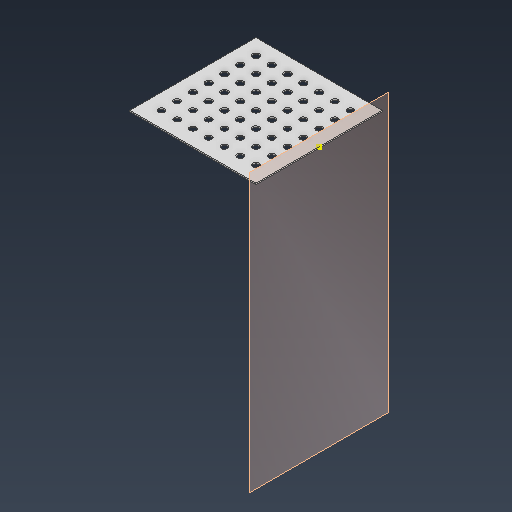
# Autodesk Inventor part: top
Saved by Autodesk Inventor 2021 (Build 250183000, 183)
## iProperties
Created: 2021-03-25
Part Number: top
Material: Generic
Document SubType Name: Modeling
Designer: noori
Density: 1 g/cm^3
Appearance: Default
Author: noori
Autodesk Inventor part; units mm, degrees
ref_plane "YZ Plane" through (0, 0, 0) normal (1, 0, 0) x (0, 1, 0)
ref_plane "XZ Plane" through (0, 0, 0) normal (0, 1, 0) x (-1, 0, 0)
ref_plane "XY Plane" through (0, 0, 0) normal (0, 0, 1) x (1, 0, 0)
sketch "Sketch1" plane through (0, 0, 0) normal (0, 1, 0) x (-1, 0, 0)
  line L0 (200, 200) -> (-200, 200)
  line L1 (-200, 200) -> (-200, -200)
  line L2 (-200, -200) -> (200, -200)
  line L3 (200, -200) -> (200, 200)
  circle A0 centre (150, 150) radius 10
  circle A1 centre (50, 50) radius 10.7206
  circle A2 centre (150, 100) radius 10
  circle A3 centre (50, 0) radius 10.7206
  circle A4 centre (50, -50) radius 10.7206
  circle A5 centre (50, -100) radius 10.7206
  circle A6 centre (50, -150) radius 10.7206
  circle A7 centre (100, 100) radius 10
  circle A8 centre (150, 50) radius 10.7206
  circle A9 centre (150, 0) radius 10.7206
  circle A10 centre (150, -50) radius 10.7206
  circle A11 centre (150, -100) radius 10.7206
  circle A12 centre (150, -150) radius 10.7206
  circle A13 centre (100, 150) radius 10
  circle A14 centre (50, 150) radius 10
  circle A15 centre (100, 50) radius 10.7206
  circle A16 centre (100, 0) radius 10.7206
  circle A17 centre (100, -50) radius 10.7206
  circle A18 centre (100, -100) radius 10.7206
  circle A19 centre (100, -150) radius 10.7206
  circle A20 centre (50, 100) radius 10
  circle A21 centre (0, 150) radius 10
  circle A22 centre (-50, 150) radius 10
  circle A23 centre (0, 100) radius 10
  circle A24 centre (-50, 100) radius 10
  circle A25 centre (0, 50) radius 10.7206
  circle A26 centre (-50, 50) radius 10.7206
  circle A27 centre (0, 0) radius 10.7206
  circle A28 centre (-0.0038, -50) radius 10.7206
  circle A29 centre (-50, 0) radius 10.7206
  circle A30 centre (0, -150) radius 10.7206
  circle A31 centre (0, -100) radius 10.7206
  circle A32 centre (-50.0026, -50) radius 10.7206
  circle A33 centre (-50.0039, -150) radius 10.7206
  circle A34 centre (-50.0039, -100) radius 10.7206
  circle A35 centre (-100, 100) radius 10
  circle A36 centre (-100, 150) radius 10
  circle A37 centre (-100, 0) radius 10
  circle A38 centre (-100.0016, -50) radius 10
  circle A39 centre (-100, 50) radius 10
  circle A40 centre (-150, 150) radius 10
  circle A41 centre (-100.0039, -100) radius 10
  circle A42 centre (-100.0039, -150) radius 10
  circle A43 centre (-150.0016, -50) radius 10
  circle A44 centre (-150.0039, -100) radius 10
  circle A45 centre (-150, 0) radius 10
  circle A46 centre (-150, 50) radius 10
  circle A47 centre (-150, 100) radius 10
  circle A48 centre (-150.0039, -150) radius 10
  point P0 (201.5875, 201.5875)
  dimension "d0" = 400
  dimension "d1" = 400
  dimension "d2" = 200
  dimension "d3" = 200
  dimension "d4" = 20
  dimension "d5" = 50
  dimension "d6" = 50
  dimension "d8" = 100
  dimension "d10" = 150
  dimension "d11" = 200
  dimension "d12" = 250
  dimension "d13" = 300
  dimension "d14" = 350
  dimension "d15" = 50
  dimension "d18" = 50
  dimension "d19" = 50
  dimension "d21" = 50
  dimension "d23" = 50
  dimension "d24" = 50
  dimension "d25" = 50
  dimension "d26" = 50
  dimension "d27" = 50
  dimension "d28" = 50
  dimension "d29" = 50
  dimension "d30" = 50
  dimension "d31" = 50
  dimension "d32" = 50
  dimension "d33" = 50
  dimension "d34" = 50
  dimension "d35" = 50
  dimension "d36" = 50
  dimension "d37" = 50
  dimension "d38" = 50
  dimension "d39" = 50
  dimension "d40" = 50
  dimension "d41" = 50
  dimension "d42" = 50
  dimension "d43" = 50
  dimension "d44" = 50
  dimension "d45" = 50
  dimension "d46" = 50
  dimension "d47" = 50
  dimension "d48" = 50
  dimension "d49" = 50.0038
  dimension "d50" = 50
  dimension "d51" = 50
  dimension "d52" = 50
  dimension "d53" = 50
  dimension "d54" = 50
  dimension "d55" = 49.9988
  dimension "d56" = 50.0039
  dimension "d57" = 50.0039
  dimension "d58" = 50
  dimension "d59" = 50
  dimension "d60" = 49.999
  dimension "d61" = 50
  dimension "d62" = 50
  dimension "d63" = 50
  dimension "d64" = 50
  dimension "d65" = 50
  dimension "d66" = 50
  dimension "d67" = 50
  dimension "d68" = 50
  dimension "d69" = 50
  constraints: 49 centre point, 8 end point, 2 parallel, 1 coincident, 1 horizontal, 1 perpendicular
  measures "d0" distance of L2.end L0.start
  measures "d1" distance of L1.end L2.end
  measures "d2" distance from line of L3 point (0, 0)
  measures "d3" distance from line of L0 point (0, 0)
  measures "d4" diameter of A0
  measures "d5" distance from line of L3 A0.centre
  measures "d6" distance from line of L0 A0.centre
  measures "d8" distance from line of L0 A2.centre
  measures "d10" distance from line of L0 A1.centre
  measures "d11" distance from line of L0 A3.centre
  measures "d12" distance from line of L0 A4.centre
  measures "d13" distance from line of L0 A5.centre
  measures "d14" distance from line of L0 A6.centre
  measures "d15" distance of A7.centre A2.centre
  measures "d18" distance of A13.centre A14.centre
  measures "d19" distance of A14.centre A21.centre
  measures "d21" distance of A21.centre A22.centre
  measures "d23" distance of A24.centre A35.centre
  measures "d24" distance of A40.centre A36.centre
  measures "d25" distance from line of L1 A40.centre
  measures "d26" distance from line of L0 A40.centre
  measures "d27" distance from line of L2 A12.centre
  measures "d28" distance of A10.centre A11.centre
  measures "d29" distance of A9.centre A10.centre
  measures "d30" distance of A8.centre A9.centre
  measures "d31" distance of A2.centre A8.centre
  measures "d32" distance of A0.centre A2.centre
  measures "d33" distance of A12.centre A11.centre
  measures "d34" distance of A0.centre A13.centre
  measures "d35" distance of A8.centre A15.centre
  measures "d36" distance of A9.centre A16.centre
  measures "d37" distance of A10.centre A17.centre
  measures "d38" distance of A11.centre A18.centre
  measures "d39" distance of A12.centre A19.centre
  measures "d40" distance of A20.centre A7.centre
  measures "d41" distance of A1.centre A15.centre
  measures "d42" distance of A3.centre A16.centre
  measures "d43" distance of A4.centre A17.centre
  measures "d44" distance of A5.centre A18.centre
  measures "d45" distance of A6.centre A19.centre
  measures "d46" distance of A23.centre A20.centre
  measures "d47" distance of A25.centre A1.centre
  measures "d48" distance of point (0, 0) A3.centre
  measures "d49" distance of A28.centre A4.centre
  measures "d50" distance of A31.centre A5.centre
  measures "d51" distance of A30.centre A6.centre
  measures "d52" distance of A24.centre A23.centre
  measures "d53" distance of A26.centre A25.centre
  measures "d54" distance of A29.centre point (0, 0)
  measures "d55" distance of A32.centre A28.centre
  measures "d56" distance of A34.centre A31.centre
  measures "d57" distance of A33.centre A30.centre
  measures "d58" distance of A39.centre A26.centre
  measures "d59" distance of A37.centre A29.centre
  measures "d60" distance of A38.centre A32.centre
  measures "d61" distance of A41.centre A34.centre
  measures "d62" distance of A42.centre A33.centre
  measures "d63" distance of A47.centre A35.centre
  measures "d64" distance of A46.centre A39.centre
  measures "d65" distance of A45.centre A37.centre
  measures "d66" distance of A43.centre A38.centre
  measures "d67" distance of A44.centre A41.centre
  measures "d68" distance of A48.centre A42.centre
  measures "d69" distance of A13.centre A7.centre
extrude "Extrusion1" add sketch "Sketch1" along normal mid plane 4
ref_plane "Work Plane1" through (200, -398, 0) normal (1, 0, 0) x (0, 0, 1)
sketch "Sketch2" plane through (200, -398, 0) normal (1, 0, 0) x (0, 0, 1)
  point P0 (0, -398)
body "Solid1"
